Motor Controller Foundation (Autodesk Fusion 360 design; units mm, degrees)
Autodesk Fusion 360 part; units mm, degrees
sketch "Sketch1" plane through (0, 0, 0) normal (0, 0, 1) x (1, 0, 0)
  line L0 (-65.475, 45.795) -> (65.475, 45.795)
  line L1 (65.475, 45.795) -> (65.475, -45.795)
  line L2 (65.475, -45.795) -> (-65.475, -45.795)
  line L3 (-65.475, -45.795) -> (-65.475, 45.795)
  dimension "d1" = 130.95
  dimension "d2" = 65.475
  dimension "d3" = 91.59
  dimension "d4" = 45.795
  constraint horizontal L0
  constraint vertical L1
  constraint horizontal L2
  constraint vertical L3
  measures "d1" distance of L1 L3
  measures "d2" distance of origin L3
  measures "d3" distance of L0 L2
  measures "d4" distance of origin L2
extrude "Extrude1" add sketch "Sketch1" along normal blind 7
sketch "Sketch2" plane through (0, 0, 7) normal (0, 0, 1) x (-1, 0, 0)
  line L0 (65.475, 45.795) -> (-65.475, 45.795)
  line L1 (-65.475, 45.795) -> (-65.475, -45.795)
  line L2 (-65.475, -45.795) -> (65.475, -45.795)
  line L3 (65.475, -45.795) -> (65.475, 45.795)
  line L4 (57.475, -43.795) -> (-57.475, -43.795)
  line L5 (-63.475, -37.795) -> (-63.475, 37.795)
  line L6 (-57.475, 43.795) -> (57.475, 43.795)
  line L7 (63.475, 37.795) -> (63.475, -37.795)
  arc A0 (57.475, -43.795) -> (63.475, -37.795) centre (57.475, -37.795) ccw
  arc A1 (63.475, 37.795) -> (57.475, 43.795) centre (57.475, 37.795) ccw
  arc A2 (-57.475, 43.795) -> (-63.475, 37.795) centre (-57.475, 37.795) ccw
  arc A3 (-63.475, -37.795) -> (-57.475, -43.795) centre (-57.475, -37.795) ccw
  dimension "d7" = 126.95
  dimension "d8" = 63.475
  dimension "d9" = 87.59
  dimension "d10" = 43.795
  dimension "d11" = 6
  constraint horizontal L4
  constraint vertical L5
  constraint horizontal L6
  constraint vertical L7
  constraint tangent L4 A0
  constraint tangent L7 A0
  constraint tangent L7 A1
  constraint tangent L6 A1
  constraint equal A0 A1
  constraint tangent L6 A2
  constraint tangent L5 A2
  constraint equal A0 A2
  constraint tangent L5 A3
  constraint tangent L4 A3
  constraint equal A0 A3
  measures "d7" distance of L5 L7
  measures "d8" distance of origin L7
  measures "d9" distance of L4 L6
  measures "d10" distance of origin L6
  measures "d11" radius of A0
fillet "Fillet2" radius 6 4 edges at (-65.475, 45.795, 3.5) (65.475, 45.795, 3.5) (65.475, -45.795, 3.5) (-65.475, -45.795, 3.5)
extrude "Extrude2" cut sketch "Sketch2" against normal blind 2 contours L4 L5 L6 L7 A0 A1 A2 A3
sketch "Sketch4" plane through (0, 0, 0) normal (0, 0, -1) x (1, 0, 0)
  arc A0 (-59.475, 45.795) -> (-65.475, 39.795) centre (-59.475, 39.795) ccw
  line L0 (-65.475, 39.795) -> (-65.475, -39.795)
  arc A1 (-65.475, -39.795) -> (-59.475, -45.795) centre (-59.475, -39.795) ccw
  line L1 (-59.475, -45.795) -> (59.475, -45.795)
  arc A2 (59.475, -45.795) -> (65.475, -39.795) centre (59.475, -39.795) ccw
  line L2 (65.475, -39.795) -> (65.475, 39.795)
  arc A3 (65.475, 39.795) -> (59.475, 45.795) centre (59.475, 39.795) ccw
  line L3 (59.475, 45.795) -> (-59.475, 45.795)
  line L4 (-68.475, 34.795) -> (-74.475, 34.795)
  line L5 (-77.475, 31.795) -> (-77.475, 25.795)
  line L6 (-74.475, 22.795) -> (-68.475, 22.795)
  line L7 (-65.475, 22.795) -> (-65.475, 34.795)
  line L8 (-68.475, -34.795) -> (-74.475, -34.795)
  line L9 (-77.475, -31.795) -> (-77.475, -25.795)
  line L10 (-74.475, -22.795) -> (-68.475, -22.795)
  line L11 (-65.475, -22.795) -> (-65.475, -34.795)
  line L12 (68.475, -34.795) -> (74.475, -34.795)
  line L13 (77.475, -31.795) -> (77.475, -25.795)
  line L14 (74.475, -22.795) -> (68.475, -22.795)
  line L15 (65.475, -22.795) -> (65.475, -34.795)
  line L16 (68.475, 34.795) -> (74.475, 34.795)
  line L17 (77.475, 31.795) -> (77.475, 25.795)
  line L18 (74.475, 22.795) -> (68.475, 22.795)
  line L19 (65.475, 22.795) -> (65.475, 34.795)
  line L20 (-65.475, 37.795) -> (-65.475, 39.795)
  line L21 (-65.475, -37.795) -> (-65.475, -39.795)
  line L22 (65.475, -37.795) -> (65.475, -39.795)
  line L23 (65.475, 37.795) -> (65.475, 39.795)
  line L24 (65.475, 19.795) -> (65.475, -19.795)
  line L25 (-65.475, -19.795) -> (-65.475, 19.795)
  arc A4 (65.475, 37.795) -> (68.475, 34.795) centre (68.475, 37.795) ccw
  arc A5 (77.475, 31.795) -> (74.475, 34.795) centre (74.475, 31.795) ccw
  arc A6 (74.475, 22.795) -> (77.475, 25.795) centre (74.475, 25.795) ccw
  arc A7 (68.475, 22.795) -> (65.475, 19.795) centre (68.475, 19.795) ccw
  arc A8 (65.475, -19.795) -> (68.475, -22.795) centre (68.475, -19.795) ccw
  arc A9 (77.475, -25.795) -> (74.475, -22.795) centre (74.475, -25.795) ccw
  arc A10 (74.475, -34.795) -> (77.475, -31.795) centre (74.475, -31.795) ccw
  arc A11 (68.475, -34.795) -> (65.475, -37.795) centre (68.475, -37.795) ccw
  arc A12 (-68.475, 34.795) -> (-65.475, 37.795) centre (-68.475, 37.795) ccw
  arc A13 (-74.475, 34.795) -> (-77.475, 31.795) centre (-74.475, 31.795) ccw
  arc A14 (-77.475, 25.795) -> (-74.475, 22.795) centre (-74.475, 25.795) ccw
  arc A15 (-65.475, 19.795) -> (-68.475, 22.795) centre (-68.475, 19.795) ccw
  arc A16 (-68.475, -22.795) -> (-65.475, -19.795) centre (-68.475, -19.795) ccw
  arc A17 (-74.475, -22.795) -> (-77.475, -25.795) centre (-74.475, -25.795) ccw
  arc A18 (-77.475, -31.795) -> (-74.475, -34.795) centre (-74.475, -31.795) ccw
  arc A19 (-65.475, -37.795) -> (-68.475, -34.795) centre (-68.475, -37.795) ccw
  dimension "d32" = 5
  dimension "d33" = 5
  dimension "d34" = 12
  dimension "d35" = 12
  dimension "d36" = 12
  dimension "d37" = 12
  dimension "d38" = 3
  dimension "d39" = 3
  dimension "d40" = 3
  dimension "d41" = 3
  constraint horizontal L4
  constraint vertical L5
  constraint horizontal L6
  constraint vertical L7
  constraint coincident L0 L7.end
  constraint horizontal L8
  constraint vertical L9
  constraint horizontal L10
  constraint vertical L11
  constraint horizontal L12
  constraint vertical L13
  constraint horizontal L14
  constraint vertical L15
  constraint horizontal L16
  constraint vertical L17
  constraint horizontal L18
  constraint vertical L19
  constraint vertical L7.end L11.end
  constraint horizontal L7.end L19.end
  constraint horizontal L11.end L15.end
  constraint vertical L15.end L19.end
  constraint vertical L2.end L19.end
  constraint coincident A0.end L0.start
  constraint coincident L0.end A1.start
  constraint coincident A2.end L2.start
  constraint coincident L2.end A3.start
  constraint coincident L19.end L23
  constraint coincident L19.end L16
  constraint tangent L23 A4
  constraint tangent L16 A4
  constraint tangent L16 A5
  constraint tangent L17 A5
  constraint equal A4 A5
  constraint tangent L17 A6
  constraint tangent L18 A6
  constraint equal A4 A6
  constraint coincident L19.start L18
  constraint coincident L19.start L24
  constraint tangent L18 A7
  constraint tangent L24 A7
  constraint equal A4 A7
  constraint coincident L15.start L24
  constraint coincident L15.start L14
  constraint tangent L24 A8
  constraint tangent L14 A8
  constraint tangent L14 A9
  constraint tangent L13 A9
  constraint equal A8 A9
  constraint tangent L13 A10
  constraint tangent L12 A10
  constraint equal A8 A10
  constraint coincident L15.end L12
  constraint coincident L15.end L22
  constraint tangent L12 A11
  constraint tangent L22 A11
  constraint equal A8 A11
  constraint coincident L7.end L20
  constraint coincident L7.end L4
  constraint tangent L20 A12
  constraint tangent L4 A12
  constraint tangent L4 A13
  constraint tangent L5 A13
  constraint equal A12 A13
  constraint tangent L5 A14
  constraint tangent L6 A14
  constraint equal A12 A14
  constraint coincident L7.start L6
  constraint coincident L7.start L25
  constraint tangent L6 A15
  constraint tangent L25 A15
  constraint equal A12 A15
  constraint coincident L11.start L25
  constraint coincident L11.start L10
  constraint tangent L25 A16
  constraint tangent L10 A16
  constraint tangent L10 A17
  constraint tangent L9 A17
  constraint equal A16 A17
  constraint tangent L9 A18
  constraint tangent L8 A18
  constraint equal A16 A18
  constraint coincident L11.end L8
  constraint coincident L11.end L21
  constraint tangent L8 A19
  constraint tangent L21 A19
  constraint equal A16 A19
  measures "d32" distance of A0.end L7.end
  measures "d33" distance of L0.end L11.end
  measures "d34" distance of L4 L6
  measures "d35" distance of L8 L10
  measures "d36" distance of L5 L7
  measures "d37" distance of L17 L19
  measures "d38" radius of A4
  measures "d39" radius of A8
  measures "d40" radius of A12
  measures "d41" radius of A16
extrude "Extrude4" add sketch "Sketch4" against normal blind 5 contours L0 L4 L5 L6 L7 A12 A13 A14 A15 | L2 L16 L17 L18 L19 A4 A5 A6 A7 | L0 L8 L9 L10 L11 A16 A17 A18 A19 | L2 L12 L13 L14 L15 A8 A9 A10 A11
sketch "Sketch5" plane through (0, 0, 5) normal (0, 0, 1) x (-1, 0, 0)
  arc A0 (-77.475, 25.795) -> (-74.475, 22.795) centre (-74.475, 25.795) ccw
  line L0 (-74.475, 22.795) -> (-68.475, 22.795)
  arc A1 (-65.475, 19.795) -> (-68.475, 22.795) centre (-68.475, 19.795) ccw
  line L1 (-65.475, 19.795) -> (-65.475, 37.795)
  arc A2 (-68.475, 34.795) -> (-65.475, 37.795) centre (-68.475, 37.795) ccw
  line L2 (-68.475, 34.795) -> (-74.475, 34.795)
  arc A3 (-74.475, 34.795) -> (-77.475, 31.795) centre (-74.475, 31.795) ccw
  line L3 (-77.475, 31.795) -> (-77.475, 25.795)
  line L4 (-68.475, -22.795) -> (-74.475, -22.795)
  line L5 (77.475, -31.795) -> (77.475, -25.795)
  point P0 (-71.475, 28.795)
  point P1 (71.475, 28.795)
  point P2 (71.475, -28.795)
  point P3 (-71.475, -28.795)
  dimension "d44" = 6
  dimension "d45" = 6
  dimension "d46" = 6
  dimension "d47" = 6
  constraint horizontal P0 P1
  constraint vertical P1 P2
  constraint horizontal P2 P3
  constraint vertical P0 P3
  measures "d44" distance of L2 P0
  measures "d45" distance of L3 P0
  measures "d46" distance of P3 L4
  measures "d47" distance of P2 L5
hole "Hole1" at (71.475, -28.795, 5) at (-71.475, -28.795, 5) at (-71.475, 28.795, 5) at (71.475, 28.795, 5) direction (0, 0, -1) diameter 3.797 depth 15 tip angle 180 countersink diameter 7.087 countersink angle 100
fillet "Fillet3" radius 3 4 edges at (-65.475, 28.795, 5) (-65.475, -28.795, 5) (65.475, -28.795, 5) (65.475, 28.795, 5)
fillet "Fillet4" radius 0.5 8 edges at (0, 43.795, 7) (61.7176, 42.0376, 7) (63.475, 0, 7) (61.7176, -42.0376, 7) (0, -43.795, 7) (-61.7176, -42.0376, 7) (-63.475, 0, 7) (-61.7176, 42.0376, 7)
sketch "Sketch6" plane through (0, 0, 5) normal (0, 0, 1) x (-1, 0, 0)
  arc A0 (-57.475, 43.795) -> (-63.475, 37.795) centre (-57.475, 37.795) ccw
  line L0 (-63.475, 37.795) -> (-63.475, -37.795)
  arc A1 (-63.475, -37.795) -> (-57.475, -43.795) centre (-57.475, -37.795) ccw
  line L1 (-57.475, -43.795) -> (57.475, -43.795)
  arc A2 (57.475, -43.795) -> (63.475, -37.795) centre (57.475, -37.795) ccw
  line L2 (63.475, -37.795) -> (63.475, 37.795)
  arc A3 (63.475, 37.795) -> (57.475, 43.795) centre (57.475, 37.795) ccw
  line L3 (57.475, 43.795) -> (-57.475, 43.795)
  point P0 (53.9745, 17.4625)
  point P1 (-53.9745, -17.4625)
  dimension "d57" = 53.9745
  dimension "d58" = 53.9745
  dimension "d61" = 17.4625
  dimension "d62" = 17.4625
  measures "d57" horizontal distance of origin P0
  measures "d58" horizontal distance of origin P1
  measures "d61" vertical distance of origin P0
  measures "d62" vertical distance of origin P1
hole "Hole2" at (53.9745, 17.4625, 5) at (-53.9745, -17.4625, 5) direction (0, 0, -1) diameter 4.85 depth 15 tip angle 180
sketch "Sketch8" plane through (0, 0, 5) normal (0, 0, 1) x (-1, 0, 0)
  circle A0 centre (-53.9745, -17.4625) radius 2.425
  circle A1 centre (53.9745, 17.4625) radius 2.425
  arc A2 (-57.475, 43.795) -> (-63.475, 37.795) centre (-57.475, 37.795) ccw
  line L0 (-63.475, 37.795) -> (-63.475, -37.795)
  arc A3 (-63.475, -37.795) -> (-57.475, -43.795) centre (-57.475, -37.795) ccw
  line L1 (-57.475, -43.795) -> (57.475, -43.795)
  arc A4 (57.475, -43.795) -> (63.475, -37.795) centre (57.475, -37.795) ccw
  line L2 (63.475, -37.795) -> (63.475, 37.795)
  arc A5 (63.475, 37.795) -> (57.475, 43.795) centre (57.475, 37.795) ccw
  line L3 (57.475, 43.795) -> (-57.475, 43.795)
  line L4 (55.975, -38.795) -> (51.5495, -38.795)
  line L5 (49.0495, -36.295) -> (49.0495, 7.5375)
  line L6 (51.5495, 10.0375) -> (55.975, 10.0375)
  line L7 (58.475, 7.5375) -> (58.475, -36.295)
  line L8 (55.975, 24.8875) -> (51.5495, 24.8875)
  line L9 (49.0495, 27.3875) -> (49.0495, 36.295)
  line L10 (51.5495, 38.795) -> (55.975, 38.795)
  line L11 (58.475, 36.295) -> (58.475, 27.3875)
  arc A6 (55.975, -38.795) -> (58.475, -36.295) centre (55.975, -36.295) ccw
  arc A7 (49.0495, -36.295) -> (51.5495, -38.795) centre (51.5495, -36.295) ccw
  arc A8 (51.5495, 10.0375) -> (49.0495, 7.5375) centre (51.5495, 7.5375) ccw
  arc A9 (58.475, 7.5375) -> (55.975, 10.0375) centre (55.975, 7.5375) ccw
  arc A10 (55.975, 24.8875) -> (58.475, 27.3875) centre (55.975, 27.3875) ccw
  arc A11 (49.0495, 27.3875) -> (51.5495, 24.8875) centre (51.5495, 27.3875) ccw
  arc A12 (51.5495, 38.795) -> (49.0495, 36.295) centre (51.5495, 36.295) ccw
  arc A13 (58.475, 36.295) -> (55.975, 38.795) centre (55.975, 36.295) ccw
  line L12 (-51.5495, -38.795) -> (-55.975, -38.795)
  line L13 (-58.475, -36.295) -> (-58.475, -27.3875)
  line L14 (-55.975, -24.8875) -> (-51.5495, -24.8875)
  line L15 (-49.0495, -27.3875) -> (-49.0495, -36.295)
  line L16 (-51.5495, -10.0375) -> (-55.975, -10.0375)
  line L17 (-58.475, -7.5375) -> (-58.475, 36.295)
  line L18 (-55.975, 38.795) -> (-51.5495, 38.795)
  line L19 (-49.0495, 36.295) -> (-49.0495, -7.5375)
  arc A14 (-51.5495, -38.795) -> (-49.0495, -36.295) centre (-51.5495, -36.295) ccw
  arc A15 (-58.475, -36.295) -> (-55.975, -38.795) centre (-55.975, -36.295) ccw
  arc A16 (-55.975, -24.8875) -> (-58.475, -27.3875) centre (-55.975, -27.3875) ccw
  arc A17 (-49.0495, -27.3875) -> (-51.5495, -24.8875) centre (-51.5495, -27.3875) ccw
  arc A18 (-51.5495, -10.0375) -> (-49.0495, -7.5375) centre (-51.5495, -7.5375) ccw
  arc A19 (-58.475, -7.5375) -> (-55.975, -10.0375) centre (-55.975, -7.5375) ccw
  arc A20 (-55.975, 38.795) -> (-58.475, 36.295) centre (-55.975, 36.295) ccw
  arc A21 (-49.0495, 36.295) -> (-51.5495, 38.795) centre (-51.5495, 36.295) ccw
  line L20 (36.2199, -38.795) -> (-36.2199, -38.795)
  line L21 (36.2199, 38.795) -> (-36.2199, 38.795)
  line L22 (44.0495, -31.8923) -> (44.0495, 31.8923)
  line L23 (-44.0495, -31.8923) -> (-44.0495, 31.8923)
  line L24 (37.5356, 35.2888) -> (1.3158, 3.6494)
  line L25 (-1.3158, 3.6494) -> (-37.5356, 35.2888)
  line L26 (-40.7337, 33.3986) -> (-4.2243, 1.5062)
  line L27 (-4.2243, -1.5062) -> (-40.7337, -33.3986)
  line L28 (-37.5356, -35.2888) -> (-1.3158, -3.6494)
  line L29 (1.3158, -3.6494) -> (37.5356, -35.2888)
  line L30 (40.7337, -33.3986) -> (4.2243, -1.5062)
  line L31 (4.2243, 1.5062) -> (40.7337, 33.3986)
  arc A22 (36.2199, -38.795) -> (37.5356, -35.2888) centre (36.2199, -36.795) ccw
  arc A23 (-37.5356, -35.2888) -> (-36.2199, -38.795) centre (-36.2199, -36.795) ccw
  arc A24 (-44.0495, -31.8923) -> (-40.7337, -33.3986) centre (-42.0495, -31.8923) ccw
  arc A25 (-40.7337, 33.3986) -> (-44.0495, 31.8923) centre (-42.0495, 31.8923) ccw
  arc A26 (-36.2199, 38.795) -> (-37.5356, 35.2888) centre (-36.2199, 36.795) ccw
  arc A27 (37.5356, 35.2888) -> (36.2199, 38.795) centre (36.2199, 36.795) ccw
  arc A28 (44.0495, 31.8923) -> (40.7337, 33.3986) centre (42.0495, 31.8923) ccw
  arc A29 (40.7337, -33.3986) -> (44.0495, -31.8923) centre (42.0495, -31.8923) ccw
  arc A30 (4.2243, 1.5062) -> (4.2243, -1.5062) centre (5.5401, 0) ccw
  arc A31 (-1.3158, 3.6494) -> (1.3158, 3.6494) centre (0, 5.1556) ccw
  arc A32 (-4.2243, -1.5062) -> (-4.2243, 1.5062) centre (-5.5401, 0) ccw
  arc A33 (1.3158, -3.6494) -> (-1.3158, -3.6494) centre (0, -5.1556) ccw
  point P0 (41.5495, -38.795)
  point P1 (-41.5495, 38.795)
  point P2 (44.0495, -36.295)
  point P3 (44.0495, 36.295)
  point P4 (0, -2.5)
  point P5 (0, 2.5)
  point P6 (-2.5, 0)
  point P7 (2.5, 0)
  dimension "d100" = 5
  dimension "d101" = 5
  dimension "d102" = 5
  dimension "d103" = 5
  dimension "d104" = 7.425
  dimension "d105" = 7.425
  dimension "d106" = 4.925
  dimension "d107" = 2.5
  dimension "d108" = 2.5
  dimension "d109" = 5
  dimension "d110" = 4.925
  dimension "d111" = 7.425
  dimension "d112" = 7.425
  dimension "d113" = 9.925
  dimension "d114" = 5
  dimension "d115" = 5
  dimension "d116" = 5
  dimension "d117" = 7.5
  dimension "d118" = 7.5
  dimension "d119" = 7.5
  dimension "d120" = 7.5
  dimension "d121" = 5
  dimension "d122" = 2.5
  dimension "d123" = 2.5
  dimension "d124" = 5
  dimension "d125" = 2
  constraint horizontal L4
  constraint vertical L5
  constraint horizontal L6
  constraint vertical L7
  constraint horizontal L8
  constraint vertical L9
  constraint horizontal L10
  constraint vertical L11
  constraint tangent L4 A6
  constraint tangent L7 A6
  constraint tangent L4 A7
  constraint tangent L5 A7
  constraint equal A6 A7
  constraint tangent L5 A8
  constraint tangent L6 A8
  constraint equal A6 A8
  constraint tangent L6 A9
  constraint tangent L7 A9
  constraint equal A6 A9
  constraint tangent L11 A10
  constraint tangent L8 A10
  constraint equal A6 A10
  constraint tangent L8 A11
  constraint tangent L9 A11
  constraint equal A6 A11
  constraint tangent L9 A12
  constraint tangent L10 A12
  constraint equal A6 A12
  constraint tangent L10 A13
  constraint tangent L11 A13
  constraint equal A6 A13
  constraint vertical A8.centre A11.centre
  constraint horizontal L12
  constraint vertical L13
  constraint horizontal L14
  constraint vertical L15
  constraint horizontal L16
  constraint vertical L17
  constraint horizontal L18
  constraint vertical L19
  constraint tangent L15 A14
  constraint tangent L12 A14
  constraint tangent L12 A15
  constraint tangent L13 A15
  constraint equal A14 A15
  constraint tangent L13 A16
  constraint tangent L14 A16
  constraint equal A14 A16
  constraint tangent L14 A17
  constraint tangent L15 A17
  constraint equal A14 A17
  constraint tangent L19 A18
  constraint tangent L16 A18
  constraint equal A14 A18
  constraint tangent L16 A19
  constraint tangent L17 A19
  constraint equal A14 A19
  constraint tangent L17 A20
  constraint tangent L18 A20
  constraint equal A14 A20
  constraint tangent L18 A21
  constraint tangent L19 A21
  constraint equal A14 A21
  constraint horizontal A7.centre A14.centre
  constraint horizontal A12.centre A21.centre
  constraint vertical A15.centre A20.centre
  constraint vertical A17.centre A18.centre
  constraint horizontal L20
  constraint horizontal L21
  constraint vertical L22
  constraint vertical L23
  constraint vertical origin P4
  constraint vertical origin P5
  constraint horizontal origin P7
  constraint horizontal origin P6
  constraint coincident P0 L29
  constraint coincident P0 L20
  constraint tangent L29 A22
  constraint tangent L20 A22
  constraint tangent L20 A23
  constraint tangent L28 A23
  constraint equal A22 A23
  constraint tangent L27 A24
  constraint tangent L23 A24
  constraint equal A22 A24
  constraint tangent L23 A25
  constraint tangent L26 A25
  constraint equal A22 A25
  constraint coincident P1 L25
  constraint coincident P1 L21
  constraint tangent L25 A26
  constraint tangent L21 A26
  constraint equal A22 A26
  constraint tangent L21 A27
  constraint tangent L24 A27
  constraint equal A22 A27
  constraint coincident P3 L31
  constraint coincident P3 L22
  constraint tangent L31 A28
  constraint tangent L22 A28
  constraint equal A22 A28
  constraint coincident P2 L22
  constraint coincident P2 L30
  constraint tangent L22 A29
  constraint tangent L30 A29
  constraint equal A22 A29
  constraint tangent L30 A30
  constraint tangent L31 A30
  constraint equal A22 A30
  constraint tangent L24 A31
  constraint tangent L25 A31
  constraint equal A22 A31
  constraint tangent L26 A32
  constraint tangent L27 A32
  constraint equal A22 A32
  constraint tangent L28 A33
  constraint tangent L29 A33
  constraint equal A22 A33
  measures "d100" distance of L2 L7
  measures "d101" distance of L2 L11
  measures "d102" distance of L3 L10
  measures "d103" distance of L1 L4
  measures "d104" distance of A1.centre L6
  measures "d105" distance of A1.centre L8
  measures "d106" distance of A1.centre L5
  measures "d107" radius of A6
  measures "d108" radius of A14
  measures "d109" distance of L0 L13
  measures "d110" distance of A0.centre L19
  measures "d111" distance of A0.centre L14
  measures "d112" distance of A0.centre L16
  measures "d113" distance of A1.centre L22
  measures "d114" distance of L19 L23
  measures "d115" distance of L1 L20
  measures "d116" distance of L3 L21
  measures "d117" distance of L5 P0
  measures "d118" distance of L1 P2
  measures "d119" distance of L3 P3
  measures "d120" distance of L19 P1
  measures "d121" distance of P4 P5
  measures "d122" distance of origin P5
  measures "d123" distance of origin P7
  measures "d124" distance of P6 P7
  measures "d125" radius of A22
extrude "Extrude6" cut sketch "Sketch8" against normal blind 5 contours L4 L5 L6 L7 A6 A7 A8 A9 | L8 L9 L10 L11 A10 A11 A12 A13 | L12 L13 L14 L15 A14 A15 A16 A17 | L16 L17 L18 L19 A18 A19 A20 A21 | L20 L28 L29 A22 A23 A33 | L21 L24 L25 A26 A27 A31 | L22 L30 L31 A28 A29 A30 | L23 L26 L27 A24 A25 A32
sketch "Sketch9" plane through (0, 0, 5) normal (0, 0, 1) x (-1, 0, 0)
  line L0 (68.3034, 27.2146) -> (68.3034, 22.7901)
  arc A0 (68.475, 22.795) -> (68.3034, 22.7901) centre (68.475, 19.795) ccw
  line L1 (68.475, 22.795) -> (74.475, 22.795)
  arc A1 (74.475, 22.795) -> (77.475, 25.795) centre (74.475, 25.795) ccw
  line L2 (77.475, 25.795) -> (77.475, 31.795)
  arc A2 (77.475, 31.795) -> (74.475, 34.795) centre (74.475, 31.795) ccw
  line L3 (74.475, 34.795) -> (68.475, 34.795)
  arc A3 (68.3034, 34.7999) -> (68.475, 34.795) centre (68.475, 37.795) ccw
  line L4 (68.3034, 34.7999) -> (68.3034, 30.3754)
  arc A4 (68.3034, 27.2146) -> (68.3034, 30.3754) centre (71.475, 28.795) ccw
  line L5 (74.475, -22.795) -> (68.475, -22.795)
  line L6 (-77.475, 31.795) -> (-77.475, 25.795)
  point P0 (71.475, 28.795)
  point P1 (71.475, -28.795)
  point P2 (-71.475, -28.795)
  point P3 (-71.475, 28.795)
  dimension "d128" = 6
  dimension "d129" = 6
  constraint coincident P0 A4.centre
  constraint vertical P0 P1
  constraint vertical P2 P3
  constraint horizontal P1 P2
  constraint horizontal P0 P3
  measures "d128" distance of P1 L5
  measures "d129" distance of P3 L6
hole "Hole3" at (-71.475, 28.795, 5) at (71.475, 28.795, 5) at (-71.475, -28.795, 5) at (71.475, -28.795, 5) direction (0, 0, 1) diameter 8 depth 5 tip angle 180
equation "d1 = 126.95 mm + 4 mm"
equation "d2 = ( 130.95 / 2 ) * 1 mm"
equation "d3 = 87.59 mm + 4 mm"
equation "d4 = ( 91.59 / 2 ) * 1 mm"
equation "d8 = ( 126.95 / 2 ) * 1 mm"
equation "d10 = ( 87.59 / 2 ) * 1 mm"
equation "d104 = ( 4.85 / 2 ) * 1 mm + 5 mm"
equation "d105 = ( 4.85 / 2 ) * 1 mm + 5 mm"
equation "d106 = ( 4.85 / 2 ) * 1 mm + 2.5 mm"
equation "d110 = ( 4.85 / 2 ) * 1 mm + 2.5 mm"
equation "d111 = ( 4.85 / 2 ) * 1 mm + 5 mm"
equation "d112 = ( 4.85 / 2 ) * 1 mm + 5 mm"
equation "d113 = ( 4.85 / 2 ) * 1 mm + 7.5 mm"
